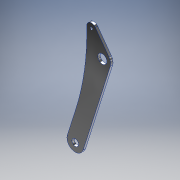
# Autodesk Inventor part: Intake Arm
Saved by Autodesk Inventor 2019.4 (Build 234330000, 330)
## iProperties
Created: 2020-01-28
Part Number: Intake Arm
Material: Aluminum 6061
Document SubType Name: Modeling
Designer: admin
Density: 2.7 g/cm^3
Appearance: Aluminum - Flat
Author: admin
Autodesk Inventor part; units mm, degrees
ref_plane "YZ Plane" through (0, 0, 0) normal (1, 0, 0) x (0, 1, 0)
ref_plane "XZ Plane" through (0, 0, 0) normal (0, 1, 0) x (-1, 0, 0)
ref_plane "XY Plane" through (0, 0, 0) normal (0, 0, 1) x (1, 0, 0)
sketch "Sketch1" plane through (0, 0, 0) normal (0, 0, 1) x (1, 0, 0)
  circle A0 centre (0, 0) radius 9.5
  arc A1 (-16.6892, 5.2651) -> (16.6892, -5.2651) centre (0, 0) ccw construction
  circle A2 centre (-57.1638, -181.1969) radius 7
  circle A3 centre (-175.4753, -121.2237) radius 88.9 construction
  circle A4 centre (-57.1638, -181.1969) radius 41.275 construction
  circle A5 centre (-57.1638, -181.1969) radius 28.5 construction
  line L0 (-263.1536, 888.7662) -> (-263.1536, -773.9924) construction
  line L1 (0, 0) -> (-57.1638, -181.1969) construction
  arc A6 (-40.4746, -186.462) -> (-73.8529, -175.9318) centre (-57.1638, -181.1969) ccw construction
  line L2 (-40.4746, -186.462) -> (16.6892, -5.2651)
  line L3 (-73.8529, -175.9318) -> (-16.6892, 5.2651)
  arc A7 (16.6892, -5.2651) -> (14.1367, 10.3153) centre (0, 0) ccw
  arc A8 (-73.8529, -175.9318) -> (-40.4746, -186.462) centre (-57.1638, -181.1969) ccw
  line L4 (0, 0) -> (263.9458, 0) construction
  circle A9 centre (-23.0802, 44.3543) radius 2.5
  circle A10 centre (-23.0802, 44.3543) radius 10
  line L5 (-23.0802, 44.3543) -> (0, 0) construction
  circle A11 centre (-30, 150) radius 2.5 construction
  line L6 (-30, 150) -> (-23.0802, 44.3543) construction
  line L7 (-16.6892, 5.2651) -> (-32.222, 40.3014)
  line L8 (-15.0021, 50.2488) -> (14.1367, 10.3153)
  arc A12 (14.1367, 10.3153) -> (-16.6892, 5.2651) centre (0, 0) ccw construction
  dimension "d0" = 19
  dimension "d1" = 35
  dimension "d4" = 14
  dimension "d5" = 177.8
  dimension "d6" = 82.55
  dimension "d7" = 57
  dimension "d8" = 190
  dimension "d9" = 35
  dimension "d10" = 107.509
  dimension "d11" = 5
  dimension "d12" = 20
  dimension "d13" = 50
  dimension "d14" = 135
  dimension "d15" = 5
  dimension "d16" = 150
  dimension "d17" = 30
  dimension "d18" = 105.8721
  constraints: 18 end point, 13 centre point, 12 point on circle, 8 tangent, 6 coincident, 1 horizontal, 1 vertical
  measures "d0" diameter of A0
  measures "d1" diameter of A1
  measures "d4" diameter of A2
  measures "d5" diameter of A3
  measures "d6" diameter of A4
  measures "d7" diameter of A5
  measures "d8" distance of L1.start L1.end
  measures "d9" diameter of A6
  measures "d10" angle of L1 L4
  measures "d11" diameter of A9
  measures "d12" diameter of A10
  measures "d13" distance of L5.start L1.start
  measures "d14" angle of L1 L5
  measures "d15" diameter of A11
  measures "d16" vertical distance of A0.centre L6.start
  measures "d17" horizontal distance of A0.centre L6.start
  measures "d18" distance of L6.start L5.start
extrude "Extrusion1" add sketch "Sketch1" along normal blind 5
fillet "Fillet1" radius 500 1 edges at (-16.6892, 5.2651, 2.5)
body "Solid1"
